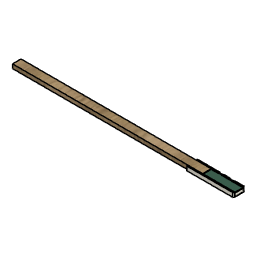
slider synth v7 (Autodesk Fusion 360 design; units mm, degrees)
Autodesk Fusion 360 part; units mm, degrees
sketch "Sketch1" plane through (0, 0, 0) normal (0, 0, 1) x (1, 0, 0)
  line L0 (0, 0) -> (-558.8, 0)
  line L1 (-558.8, 0) -> (-558.8, 25)
  line L2 (-558.8, 25) -> (0, 25)
  line L3 (0, 25) -> (0, 0)
  dimension "d1" = 25
  dimension "d2" = 558.8
  constraint horizontal L0
  constraint vertical L1
  constraint horizontal L2
  constraint vertical L3
  constraint coincident L0.start L3.end
  measures "d1" distance of L0.start L2.end
  measures "d2" distance of L0.start L0.end
extrude "Extrude1" add sketch "Sketch1" along normal blind 12 makes body 1
sketch "Sketch2" plane through (0, 0, 0) normal (0, 0, -1) x (1, 0, 0)
  line L0 (-558.8, -25) -> (0, -25)
  line L1 (0, -25) -> (0, 0)
  line L2 (0, 0) -> (-558.8, 0)
  line L3 (-558.8, 0) -> (-558.8, -25)
  line L4 (-45, 0) -> (-45, -25)
  line L5 (-45, -25) -> (0, -25)
  line L6 (0, -25) -> (0, 0)
  line L7 (-45, 0) -> (-45, 4)
  line L8 (-45, 4) -> (95, 4)
  line L9 (95, 4) -> (95, -29)
  line L10 (95, -29) -> (-45, -29)
  line L11 (-45, -29) -> (-45, -25)
  line L12 (-45, 0) -> (0, 0)
  line L13 (-45, 0.15) -> (0.15, 0.15)
  line L14 (0.15, -25.15) -> (0.15, 0.15)
  line L15 (-45, -25.15) -> (0.15, -25.15)
  line L16 (0.15, -20) -> (-90.15, -20)
  line L17 (-90.15, -20) -> (-90.15, -5)
  line L18 (-90.15, -5) -> (0.15, -5)
  line L19 (0.15, -5) -> (0.15, -20)
  line L20 (0.15, -20) -> (-90.15, -5) construction
  line L21 (-90.15, -20) -> (0.15, -5) construction
  line L22 (-40, -25.15) -> (-40, 0.15)
  point P0 (-45, -12.5)
  dimension "d5" = 45
  dimension "d6" = 4
  dimension "d8" = -0.15
  dimension "d9" = 140
  dimension "d12" = 5
  dimension "d38" = 5
  constraint vertical L4
  constraint horizontal L5
  constraint vertical L6
  constraint coincident L0 L4.end
  constraint coincident L1.end L2.start
  constraint perpendicular L2 L7
  constraint perpendicular L4 L8
  constraint perpendicular L8 L9
  constraint perpendicular L9 L10
  constraint perpendicular L5 L11
  constraint perpendicular L1 L12
  constraint horizontal L16
  constraint perpendicular L16 L17
  constraint parallel L16 L18
  constraint parallel L17 L19
  constraint coincident L20 P0
  constraint coincident L21 P0
  constraint midpoint L4 P0
  constraint coincident L14 L16.start
  constraint coincident L15 L22.start
  constraint coincident L13 L22.end
  constraint perpendicular L13 L22
  measures "d5" distance of L1.end L4.start
  measures "d6" distance of L4.end L10.end
  measures "d9" distance of L9.end L10.end
  measures "d12" distance of L5 L16
  measures "d38" distance of L4 L22
extrude "Extrude19" add sketch "Sketch2" against normal blind 12 separate body contours L7 L8 L9 L10 L11 L13 L14 L15 L19 makes body 2
sketch "Sketch10" plane through (0, 0, 12) normal (0, 0, 1) x (-1, 0, 0)
  line L0 (-0.15, 0.15) -> (45, 0.15)
  line L1 (45, 0.15) -> (45, 4)
  line L2 (45, 4) -> (-95, 4)
  line L3 (-95, 4) -> (-95, -29)
  line L4 (-95, -29) -> (45, -29)
  line L5 (45, -29) -> (45, -25.15)
  line L6 (45, -25.15) -> (-0.15, -25.15)
  line L7 (-0.15, -25.15) -> (-0.15, 0.15)
  line L8 (-0.15, 0.15) -> (-95, 0.15)
  line L9 (-95, 0.15) -> (-95, -25.15)
  line L10 (-95, -25.15) -> (-0.15, -25.15)
  line L11 (-0.15, -25.15) -> (-0.15, 0.15)
  constraint horizontal L8
  constraint vertical L9
  constraint horizontal L10
  constraint vertical L11
  constraint coincident L3 L9.end
  constraint coincident L0.start L7.end
extrude "Extrude20" cut sketch "Sketch10" against normal blind 1.8 contours L3 L7 L8 L9 L10 L11 bodies 2
sketch "Sketch12" plane through (0, 0, 10.2) normal (0, 0, 1) x (-1, 0, 0)
  line L0 (-0.15, -25.15) -> (-0.15, 0.15)
  line L1 (-0.15, 0.15) -> (-95, 0.15)
  line L2 (-95, 0.15) -> (-95, -25.15)
  line L3 (-95, -25.15) -> (-0.15, -25.15)
  line L4 (-0.3, 0) -> (-94.85, 0)
  line L5 (-94.85, 0) -> (-94.85, -25)
  line L6 (-94.85, -25) -> (-0.3, -25)
  line L7 (-0.3, -25) -> (-0.3, 0)
  dimension "d98" = -0.15
extrude "Extrude22" add sketch "Sketch12" along normal blind 1.6 from surface at 0.2 separate body contours L4 L5 L6 L7 makes body 3
sketch "Sketch11" plane through (0, 0, 10.2) normal (0, 0, 1) x (-1, 0, 0)
  line L0 (-0.15, -25.15) -> (-0.15, 0.15)
  line L1 (-0.15, 0.15) -> (-95, 0.15)
  line L2 (-95, 0.15) -> (-95, -25.15)
  line L3 (-95, -25.15) -> (-0.15, -25.15)
  line L4 (-47.575, -25.15) -> (-47.575, 0.15) construction
  line L5 (-95, -12.5) -> (-47.575, -12.5) construction
  line L6 (-93, -23.15) -> (-2.15, -23.15)
  line L7 (-2.15, -23.15) -> (-2.15, -1.85)
  line L8 (-2.15, -1.85) -> (-93, -1.85)
  line L9 (-93, -1.85) -> (-93, -23.15)
  line L10 (-93, -23.15) -> (-2.15, -1.85) construction
  line L11 (-2.15, -23.15) -> (-93, -1.85) construction
  point P0 (-47.575, -12.5)
  dimension "d93" = 2
  dimension "d94" = 2
  constraint midpoint L3 L4.start
  constraint midpoint L1 L4.end
  constraint midpoint L2 L5.start
  constraint midpoint L4 P0
  constraint horizontal L6
  constraint perpendicular L6 L7
  constraint parallel L6 L8
  constraint parallel L7 L9
  constraint coincident L10 P0
  constraint coincident L11 P0
  constraint coincident P0 L5.end
  measures "d93" distance of L2 L9
  measures "d94" distance of L1 L8
extrude "Extrude21" cut sketch "Sketch11" against normal blind 8 contours L6 L7 L8 L9 bodies 2
sketch "Sketch13" plane through (0, 0, 12) normal (0, 0, 1) x (-1, 0, 0)
  line L0 (-0.3, -25) -> (-0.3, 0)
  line L1 (-0.3, 0) -> (-94.85, 0)
  line L2 (-94.85, 0) -> (-94.85, -25)
  line L3 (-94.85, -25) -> (-0.3, -25)
sketch "Sketch15" plane through (0, 0, 10.2) normal (0, 0, 1) x (-1, 0, 0)
  line L0 (-2.15, -23.15) -> (-93, -23.15)
  line L1 (-93, -23.15) -> (-93, -1.85)
  line L2 (-93, -1.85) -> (-2.15, -1.85)
  line L3 (-2.15, -1.85) -> (-2.15, -23.15)
  line L4 (-0.15, -25.15) -> (-0.15, 0.15)
  line L5 (-0.15, 0.15) -> (-95, 0.15)
  line L6 (-95, 0.15) -> (-95, -25.15)
  line L7 (-95, -25.15) -> (-0.15, -25.15)
  line L8 (-0.15, -25.15) -> (-23.15, -25.15)
  line L9 (-23.15, -25.15) -> (-31.65, -25.15)
  line L10 (-23.15, -25.15) -> (-31.65, -25.15)
  line L11 (-31.65, -25.15) -> (-31.65, -23.15)
  line L12 (-31.65, -23.15) -> (-23.15, -23.15)
  line L13 (-23.15, -23.15) -> (-23.15, -25.15)
  line L14 (-31.65, -25.15) -> (-51.65, -25.15)
  line L15 (-51.65, -25.15) -> (-63.65, -25.15)
  dimension "d102" = 23
  dimension "d103" = 8.5
  dimension "d106" = 20
  dimension "d107" = 12
  constraint coincident L4.start L7.end
  constraint perpendicular L4 L8
  constraint parallel L7 L9
  constraint horizontal L10
  constraint vertical L11
  constraint horizontal L12
  constraint vertical L13
  constraint coincident L0 L11.end
  constraint perpendicular L11 L14
  constraint parallel L7 L15
  measures "d102" distance of L4.start L8.end
  measures "d103" distance of L8.end L9.end
  measures "d106" distance of L9.end L14.end
  measures "d107" distance of L14.end L15.end
extrude "Extrude23" cut sketch "Sketch15" against normal blind 4 contours L0 L7 L9 L10 L11 L12 L13 bodies 2
sketch "Sketch16" plane through (0, 25.15, 0) normal (0, -1, 0) x (1, 0, 0)
  line L0 (-45, 0) -> (0.15, 0)
  line L1 (0.15, 0) -> (0.15, 10.2)
  line L2 (0.15, 10.2) -> (23.15, 10.2)
  line L3 (23.15, 10.2) -> (23.15, 6.2)
  line L4 (23.15, 6.2) -> (31.65, 6.2)
  line L5 (31.65, 6.2) -> (31.65, 10.2)
  line L6 (31.65, 10.2) -> (95, 10.2)
  line L7 (95, 10.2) -> (95, 12)
  line L8 (95, 12) -> (-45, 12)
  line L9 (-45, 12) -> (-45, 0)
  line L10 (31.65, 10.2) -> (51.65, 10.2)
  line L11 (51.65, 10.2) -> (63.65, 10.2)
  line L12 (51.65, 10.2) -> (63.65, 10.2)
  line L13 (63.65, 10.2) -> (63.65, 12)
  line L14 (63.65, 12) -> (51.65, 12)
  line L15 (51.65, 12) -> (51.65, 10.2)
  line L16 (31.65, 10.2) -> (23.15, 10.2)
  line L17 (23.15, 10.2) -> (23.15, 12)
  line L18 (23.15, 12) -> (31.65, 12)
  line L19 (31.65, 12) -> (31.65, 10.2)
  dimension "d108" = 20
  dimension "d109" = 12
  constraint coincident L5.end L6.start
  constraint perpendicular L5 L10
  constraint parallel L6 L11
  constraint horizontal L12
  constraint vertical L13
  constraint horizontal L14
  constraint vertical L15
  constraint coincident L8 L13.end
  constraint horizontal L16
  constraint vertical L17
  constraint horizontal L18
  constraint vertical L19
  constraint coincident L8 L17.end
  measures "d108" distance of L5.end L10.end
  measures "d109" distance of L10.end L11.end
extrude "Extrude24" cut sketch "Sketch16" against normal blind 17.39 contours L8 L16 L17 L18 L19 | L6 L8 L11 L12 L13 L14 L15 bodies 2
fillet "Fillet1" radius 3 4 edges at (-45, -4, 6) (95, -4, 6) (95, 29, 6) (-45, 29, 6) on bodies 2
fillet "Fillet2" radius 0.5 4 edges at (31.65, 27.075, 10.2) (63.65, 27.075, 10.2) (23.15, 27.075, 10.2) (51.65, 27.075, 10.2) on bodies 2
named bodies: "Plywood", "Case", "PCB"
